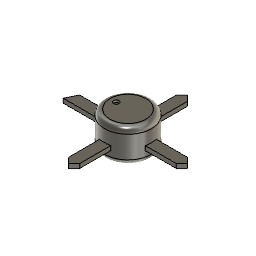
ATF-26884 (Autodesk Fusion 360 design; units mm, degrees)
part number: 2026-08-09-18-36-20-229
Autodesk Fusion 360 part; units mm, degrees
sketch "Sketch1" plane through (0, 0, 0) normal (0, 0, 1) x (1, 0, 0)
  circle A0 centre (0, 0) radius 1.075
  dimension "d1" = 2.15
  constraint coincident A0.centre origin
  measures "d1" diameter of A0
extrude "Extrude1" add sketch "Sketch1" along normal blind 0.51
sketch "Sketch2" plane through (0, 0, 0.51) normal (0, 0, 1) x (-1, 0, 0)
  circle A0 centre (0, 0) radius 1.075
  line L0 (0, 0) -> (-1.075, 0) construction
  line L1 (0, 0) -> (-2.73, 0) construction
  line L2 (0, 0) -> (2.73, 0) construction
  line L3 (2.73, 0.255) -> (2.73, -0.255) construction
  line L4 (0, -2.73) -> (0, -2.73)
  line L5 (0, -2.73) -> (0.255, -2.475)
  line L6 (-0.255, -2.475) -> (0, -2.73)
  line L7 (-0.255, 2.475) -> (0, 2.73)
  line L8 (0, 2.73) -> (0.255, 2.475)
  line L9 (-2.475, -0.255) -> (-2.73, 0)
  line L10 (-2.73, 0) -> (-2.475, 0.255)
  line L11 (2.73, 0.255) -> (2.475, 0.255) construction
  line L12 (2.475, 0.255) -> (2.475, -0.255) construction
  line L13 (2.475, -0.255) -> (2.73, 0.255)
  arc A1 (-1.0443, -0.255) -> (-0.255, -1.0443) centre (0, 0) ccw
  arc A2 (0.255, -1.0443) -> (1.0443, -0.255) centre (0, 0) ccw
  arc A3 (-0.255, 1.0443) -> (-1.0443, 0.255) centre (0, 0) ccw
  arc A4 (1.0443, 0.255) -> (0.255, 1.0443) centre (0, 0) ccw
  line L14 (2.475, -0.255) -> (1.0443, -0.255)
  line L15 (-1.0443, -0.255) -> (-2.475, -0.255)
  line L16 (0.255, 2.475) -> (0.255, 1.0443)
  line L17 (0.255, -1.0443) -> (0.255, -2.475)
  line L18 (0.255, 2.475) -> (0.255, 1.0443)
  line L19 (0.255, -1.0443) -> (0.255, -2.475)
  line L20 (-0.255, -2.475) -> (-0.255, -1.0443)
  line L21 (-0.255, -2.475) -> (-0.255, -1.0443)
  line L22 (-2.475, 0.255) -> (-1.0443, 0.255)
  line L23 (1.0443, 0.255) -> (2.73, 0.255)
  line L24 (-0.255, 1.0443) -> (-0.255, 2.475)
  line L25 (-0.255, 1.0443) -> (-0.255, 2.475)
  point P0 (-2.73, -0.255)
  dimension "d4" = 2.73
  dimension "d5" = 2.73
  dimension "d6" = 0.51
  dimension "d8" = 0.51
  dimension "d21" = 0.255
  constraint coincident A0.centre L0.start
  constraint coincident A0 L0.end
  constraint horizontal L0
  constraint parallel L0 L1
  constraint parallel L0 L2
  constraint midpoint L2.end L3
  constraint perpendicular L2 L3
  constraint coincident L4 L6.start
  constraint coincident P0 L15
  constraint perpendicular L3 L11
  constraint perpendicular L12 L14
  constraint coincident A0 A1.end
  constraint coincident A0 A2.end
  constraint coincident A0 A3.end
  constraint coincident A0 A4.start
  constraint collinear L14 L15
  constraint collinear L16 L17
  constraint collinear L18 L19
  constraint collinear L22 L23
  measures "d4" distance of A0.centre L1.end
  measures "d5" distance of A0.centre L2.end
  measures "d6" distance of L3.start L3.end
  measures "d8" distance of L3.end L3.start
  measures "d21" distance of L3.start L11.end
extrude "Extrude2" add sketch "Sketch2" along normal blind 0.2
sketch "Sketch3" plane through (0, 0, 0.71) normal (0, 0, 1) x (-1, 0, 0)
  arc A0 (-1.0443, -0.255) -> (-0.255, -1.0443) centre (0, 0) ccw
  line L0 (-0.255, -1.0443) -> (-0.255, -2.475)
  line L1 (-0.255, -2.475) -> (0, -2.73)
  line L2 (0, -2.73) -> (0.255, -2.475)
  line L3 (0.255, -2.475) -> (0.255, -1.0443)
  arc A1 (0.255, -1.0443) -> (1.0443, -0.255) centre (0, 0) ccw
  line L4 (1.0443, -0.255) -> (2.475, -0.255)
  line L5 (2.475, -0.255) -> (2.73, 0.255)
  line L6 (2.73, 0.255) -> (1.0443, 0.255)
  arc A2 (1.0443, 0.255) -> (0.255, 1.0443) centre (0, 0) ccw
  line L7 (0.255, 1.0443) -> (0.255, 2.475)
  line L8 (0.255, 2.475) -> (0, 2.73)
  line L9 (0, 2.73) -> (-0.255, 2.475)
  line L10 (-0.255, 2.475) -> (-0.255, 1.0443)
  arc A3 (-0.255, 1.0443) -> (-1.0443, 0.255) centre (0, 0) ccw
  line L11 (-1.0443, 0.255) -> (-2.475, 0.255)
  line L12 (-2.475, 0.255) -> (-2.73, 0)
  line L13 (-2.73, 0) -> (-2.475, -0.255)
  line L14 (-2.475, -0.255) -> (-1.0443, -0.255)
  circle A4 centre (0, 0) radius 1.075
  constraint concentric A0 A4
extrude "Extrude3" add sketch "Sketch3" along normal blind 0.81 contours A0 A1 A2 A3 A4
fillet "Fillet1" radius 0.25 1 edges at (1.0023, 0.3887, 1.52)
fillet "Fillet2" radius 0.25 1 edges at (-1.0023, -0.3887, 0)
sketch "Sketch4" plane through (0, 0, 1.52) normal (0, 0, 1) x (-1, 0, 0)
  circle A0 centre (0, 0) radius 0.825
  line L0 (0, 0) -> (0.5375, 0) construction
  circle A1 centre (0.5375, 0) radius 0.125
  dimension "d30" = 0.5375
  dimension "d31" = 0.25
  constraint coincident A0.centre L0.start
  constraint horizontal L0
  constraint coincident L0.end A1.centre
  measures "d30" distance of A0.centre L0.end
  measures "d31" diameter of A1
extrude "Extrude4" cut sketch "Sketch4" against normal blind 0.1 contours A1
